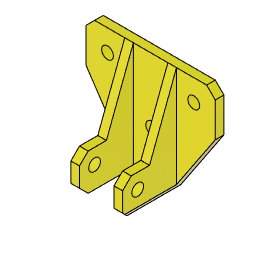
Idler Top Rear Buddy_1x (Autodesk Fusion 360 design; units mm, degrees)
Autodesk Fusion 360 part; units mm, degrees
sketch "Sketch1" plane through (0, 0, 0) normal (0, 1, 0) x (1, 0, 0)
  line L0 (-30, -20) -> (30, -20)
  line L1 (30, -20) -> (30, 0)
  line L2 (30, 0) -> (-30, 0)
  line L3 (-30, 0) -> (-30, -20)
  line L4 (-10, 0) -> (-10, 30)
  line L5 (-10, 30) -> (10, 30)
  line L6 (10, 30) -> (10, 0)
  line L7 (0, 0) -> (0, 30) construction
  line L8 (-30, 0) -> (-10, 30)
  line L9 (10, 30) -> (30, 0)
  point P0 (-10, 0)
  dimension "d5947" = 60
  dimension "d5948" = 20
  dimension "d5953" = 20
  dimension "d5954" = 30
  dimension "d6086" = 0
  dimension "d6087" = 0
  dimension "d6088" = 0
  dimension "d6089" = 0
  dimension "d6114" = 0
  dimension "d6115" = 0
  dimension "d6116" = 0
  dimension "d6117" = 0
  dimension "d6126" = 0
  dimension "d6127" = 0
  dimension "d6128" = 0
  dimension "d6129" = 0
  dimension "d6150" = 0
  dimension "d6151" = 0
  dimension "d6152" = 0
  dimension "d6153" = 0
  dimension "d6182" = 0
  dimension "d6183" = 0
  dimension "d6184" = 0
  dimension "d6185" = 0
  dimension "d6319" = 0
  dimension "d6320" = 0
  dimension "d6321" = 0
  dimension "d6322" = 0
  dimension "d6335" = 0
  dimension "d6336" = 0
  dimension "d6337" = 0
  dimension "d6338" = 0
  dimension "d53" = 0
  dimension "d54" = 0
  dimension "d55" = 0
  dimension "d56" = 0
  dimension "d65" = 0
  dimension "d66" = 0
  dimension "d67" = 0
  dimension "d68" = 0
  dimension "d220" = 0
  dimension "d221" = 0
  dimension "d222" = 0
  dimension "d223" = 0
  constraint horizontal L0
  constraint vertical L1
  constraint horizontal L2
  constraint vertical L3
  constraint midpoint L2 L7.start
  constraint coincident L2 P0
  constraint perpendicular L2 L4
  constraint perpendicular L4 L5
  constraint coincident L2 L6.end
  constraint perpendicular L2 L6
  constraint coincident L7.start origin
  constraint perpendicular L5 L7
  constraint midpoint L5 L7.end
  measures "d5947" distance of L0.start L0.end
  measures "d5948" distance of L0.start L2.end
  measures "d5953" distance of L4.end L5.end
  measures "d5954" distance of L5.end L6.end
extrude "Extrude1" add sketch "Sketch1" along normal blind 4
sketch "Sketch6" plane through (0, 4, 0) normal (0, 1, 0) x (-1, 0, 0)
  line L0 (30, 0) -> (30, 20)
  line L1 (30, 20) -> (-30, 20)
  line L2 (-30, 20) -> (-30, 0)
  line L3 (-30, 0) -> (-10, -30)
  line L4 (-10, -30) -> (10, -30)
  line L5 (10, -30) -> (30, 0)
  line L6 (-12, -13) -> (12, -13)
  line L7 (12, -13) -> (12, -30)
  line L8 (12, -30) -> (-10, -30)
  line L9 (-12, -27) -> (-12, -13)
  line L10 (0, -13) -> (0, 20)
  line L11 (8, -13) -> (8, -30)
  line L12 (-8, -30) -> (-8, -13)
  dimension "d6300" = 14
  dimension "d6301" = 16
  dimension "d154" = 4
  constraint horizontal L6
  constraint vertical L7
  constraint horizontal L8
  constraint vertical L9
  constraint coincident L4 L7.end
  constraint midpoint L6 L10.start
  constraint perpendicular L1 L10
  constraint midpoint L1 L10.end
  constraint coincident L6 L11.start
  constraint perpendicular L8 L11
  constraint coincident L8 L12.start
  constraint coincident L6 L12.end
  constraint perpendicular L6 L12
  constraint symmetric L10 L11.start L12.end
  constraint coincident L8 L11.end
  constraint coincident L3 L9.start
  measures "d6300" distance of L6.start L9.start
  measures "d6301" distance of L11 L12
  measures "d154" distance of L7 L11
extrude "Extrude9" add sketch "Sketch6" along normal blind 25 contours L4 L5 L6 L7 L8 L11 | L3 L4 L6 L8 L9 L12
hole "Hole6" at (12, 22, -20) direction (-1, 0, 0) diameter 5.5 depth 55 tip angle 118
sketch "Sketch7" plane through (12, 0, 0) normal (1, 0, 0) x (0, 1, 0)
  circle A0 centre (22, -20) radius 2.75
  line L0 (4, -13) -> (4, -27)
  line L1 (29, -27) -> (29, -13)
  line L2 (29, -13) -> (4, -13)
  circle A1 centre (22, -20) radius 2.75
  line L3 (4, -13) -> (29, -13)
  line L4 (29, -27) -> (29, -13)
  line L5 (4, -13) -> (4, 0)
  line L6 (4, 0) -> (4, 20)
  line L7 (0, 0) -> (0, -30)
  line L8 (0, -30) -> (29, -30)
  line L9 (0, 20) -> (4, 20)
  line L10 (0, 0) -> (0, 20)
  line L11 (4, 20) -> (16.5, -13)
  line L12 (4, -27) -> (29, -27)
  line L13 (29, -30) -> (29, -27)
  constraint coincident L6.end L9.end
  constraint coincident L3 L11.end
  constraint midpoint L3 L11.end
extrude "Extrude10" add sketch "Sketch7" against normal blind 4 contours L2 L3 L5 L6 L11
ref_plane "WorkPlane2" through (0, 2, 10) normal (1, 0, 0) x (0, 0, -1)
hole "Hole7" at (20, 4, 10) direction (0, -1, 0) diameter 5.5 depth 55 tip angle 118
mirror "Mirror1" about plane through (0, 2, 10) normal (1, 0, 0) of "Extrude10", "Hole7"
hole "Hole8" at (-0.5, 4, -10) direction (0, -1, 0) diameter 5.5 depth 55 tip angle 118
chamfer "Chamfer5" distance 4 angle 45 6 edges at (30, 2, 20) (-30, 2, 20) (-9, 29, -30) (9, 29, -30) (-10, 29, -13) (10, 29, -13)
equation "d6301 = 12 mm + 4 mm"
named bodies: "11mm Idler Top Rear Buddy_1x_SN_BN"
